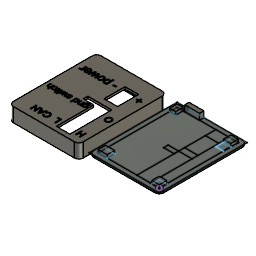
CANbuttonPresser (Autodesk Fusion 360 design; units mm, degrees)
Autodesk Fusion 360 part; units mm, degrees
sketch "Sketch1" plane through (0, 0, 0) normal (0, 0, 1) x (1, 0, 0)
  line L0 (0, 0) -> (-41, 0)
  line L1 (-41, 0) -> (-41, 53)
  line L2 (-41, 53) -> (0, 53)
  line L3 (0, 53) -> (0, 0)
  line L4 (-44, -3) -> (-44, 56)
  line L5 (-44, 56) -> (3, 56)
  line L6 (3, 56) -> (3, -3)
  line L7 (3, -3) -> (-44, -3)
  line L8 (-36, 53) -> (-26, 53)
  line L9 (-26, 53) -> (-26, 56)
  line L10 (-26, 56) -> (-36, 56)
  line L11 (-36, 56) -> (-36, 53)
  line L12 (-6, 53) -> (-6, 0)
  line L13 (-15, 53) -> (-15, 0)
  line L14 (-15, 28) -> (-22, 28)
  line L15 (-22, 28) -> (-22, 25)
  line L16 (-22, 25) -> (-15, 25)
  line L17 (-15, 25) -> (-15, 28) construction
  line L18 (-35, 0) -> (-41, 0)
  line L19 (-41, 0) -> (-41, 5)
  line L20 (-41, 5) -> (-35, 5)
  line L21 (-35, 5) -> (-35, 0)
  line L22 (-41, 53) -> (-37, 53)
  line L23 (-37, 53) -> (-37, 48)
  line L24 (-37, 48) -> (-41, 48)
  line L25 (-41, 48) -> (-41, 53)
  line L26 (0, 53) -> (-5, 53)
  line L27 (-5, 53) -> (-5, 48)
  line L28 (-5, 48) -> (0, 48)
  line L29 (0, 48) -> (0, 53)
  line L30 (0, 0) -> (-5, 0)
  line L31 (-5, 0) -> (-5, 5)
  line L32 (-5, 5) -> (0, 5)
  line L33 (0, 5) -> (0, 0)
  line L34 (-15, 46) -> (-6, 46)
  line L35 (-15, 28) -> (-6, 28)
  line L36 (-15, 32) -> (-6, 32)
  line L37 (-5, 48) -> (0, 48)
  line L38 (0, 48) -> (0, 43)
  line L39 (0, 43) -> (-5, 43)
  line L40 (-5, 43) -> (-5, 48)
  dimension "d1" = 53
  dimension "d2" = 41
  dimension "d3" = -3
  dimension "d4" = 10
  dimension "d5" = 5
  dimension "d6" = 6
  dimension "d7" = 9
  dimension "d8" = 25
  dimension "d9" = 7
  dimension "d10" = 3
  dimension "d21" = 7
  dimension "d32" = 4
  dimension "d41" = 4
  constraint horizontal L0
  constraint vertical L1
  constraint horizontal L2
  constraint vertical L3
  constraint coincident L0.start L3.end
  constraint horizontal L8
  constraint vertical L9
  constraint horizontal L10
  constraint vertical L11
  constraint coincident L2 L8.start
  constraint coincident L2 L12.start
  constraint coincident L0 L12.end
  constraint perpendicular L0 L12
  constraint coincident L2 L13.start
  constraint coincident L0 L13.end
  constraint perpendicular L0 L13
  constraint horizontal L14
  constraint vertical L15
  constraint horizontal L16
  constraint vertical L17
  constraint coincident L13 L14.start
  constraint horizontal L18
  constraint vertical L19
  constraint horizontal L20
  constraint vertical L21
  constraint coincident L1 L19.end
  constraint horizontal L22
  constraint vertical L23
  constraint horizontal L24
  constraint vertical L25
  constraint horizontal L26
  constraint vertical L27
  constraint horizontal L28
  constraint vertical L29
  constraint horizontal L30
  constraint vertical L31
  constraint horizontal L32
  constraint vertical L33
  constraint coincident L13 L34.start
  constraint coincident L12 L34.end
  constraint perpendicular L12 L34
  constraint coincident L12 L35.end
  constraint perpendicular L12 L35
  constraint coincident L13 L36.start
  constraint coincident L12 L36.end
  constraint perpendicular L12 L36
  constraint horizontal L37
  constraint vertical L38
  constraint horizontal L39
  constraint vertical L40
  constraint coincident L3 L38.end
  measures "d1" distance of L0.end L1.end
  measures "d2" distance of L0.start L0.end
  measures "d4" distance of L8.start L8.end
  measures "d5" distance of L1.end L11
  measures "d6" distance of L3 L12
  measures "d7" distance of L12 L13
  measures "d8" distance of L2 L14
  measures "d9" distance of L14.start L14.end
  measures "d10" distance of L14.end L15.end
  measures "d21" distance of L2 L34
  measures "d32" distance of L35 L36
  measures "d41" distance of L23.end L24.end
extrude "Extrude1" add sketch "Sketch1" along normal blind 1.5 contours L0 L1 L2 L3 L4 L5 L6 L7 L9 L11 L18 L19 L22 L25 L26 L29 L30 L33 L38 | L0 L3 L30 L31 L32 L33 | L0 L2 L3 L12 L27 L31 L32 L39 L40 | L3 L28 L37 L38 L39 L40 | L0 L1 L2 L8 L13 L14 L15 L16 L20 L21 L23 L24 | L12 L13 L35 L36 | L2 L3 L26 L27 L28 L29 L37 | L0 L1 L18 L19 L20 L21 | L2 L12 L13 L34 | L1 L2 L22 L23 L24 L25 | L2 L5 L8 L9 L10 L11 makes body 1
extrude "Extrude2" add sketch "Sketch1" against normal blind 8 contours L0 L1 L2 L3 L4 L5 L6 L7 L9 L11 L18 L19 L22 L25 L26 L29 L30 L33 L38 bodies 1
extrude "Extrude7" add sketch "Sketch1" against normal blind 3 contours L0 L3 L30 L31 L32 L33 | L3 L28 L37 L38 L39 L40 | L0 L1 L18 L19 L20 L21 bodies 1
move_body "Move1" bodies 1 to x (1, 0, 0) y (0, 1, 0) z (0, 0, 1) at (-54, 0, 0)
extrude "Extrude8" add sketch "Sketch1" against normal blind 1.2 separate body makes body 2
extrude "Extrude4" add sketch "Sketch1" along normal blind 2 and the other way blind 1 contours L0 L3 L30 L31 L32 L33 | L2 L3 L26 L27 L28 L29 L37 | L0 L1 L18 L19 L20 L21 | L1 L2 L22 L23 L24 L25 bodies 2
extrude "Extrude5" add sketch "Sketch1" along normal blind 4 contours L2 L5 L8 L9 L10 L11 bodies 2
fillet "Fillet1" radius 2 2 edges at (-80, 54.5, 0) (-90, 54.5, 0) on bodies 1
fillet "Fillet2" radius 3 8 edges at (-51, 56, -3.25) (-51, -3, -3.25) (-98, 56, -3.25) (-98, -3, -3.25) (3, -3, -0.6) (-44, -3, -0.6) (3, 56, -0.6) (-44, 56, -0.6) on bodies 1 2
sketch "Sketch2" plane through (0, 0, 1.5) normal (0, 0, 1) x (-1, 0, 0)
  arc A0 (98, 0) -> (95, 3) centre (95, 0) ccw
  line L0 (95, 3) -> (54, 3)
  arc A1 (54, 3) -> (51, 0) centre (54, 0) ccw
  line L1 (51, 0) -> (51, -53)
  arc A2 (51, -53) -> (54, -56) centre (54, -53) ccw
  line L2 (54, -56) -> (95, -56)
  arc A3 (95, -56) -> (98, -53) centre (95, -53) ccw
  line L3 (98, -53) -> (98, 0)
  line L4 (54.5628, -46.0404) -> (98.0169, -45.7556) construction
  line L5 (98.0169, -45.7556) -> (97.9831, -40.5942) construction
  line L6 (97.9831, -40.5942) -> (54.529, -40.8791) construction
  line L7 (54.529, -40.8791) -> (54.5628, -46.0404) construction
  line L8 (53.3651, -24.4416) -> (96.8192, -24.1567) construction
  line L9 (96.8192, -24.1567) -> (96.7854, -18.9954) construction
  line L10 (96.7854, -18.9954) -> (53.3313, -19.2803) construction
  line L11 (53.3313, -19.2803) -> (53.3651, -24.4416) construction
  line L12 (54.8378, -6.9343) -> (98.292, -6.6494) construction
  line L13 (98.292, -6.6494) -> (98.2581, -1.4881) construction
  line L14 (98.2581, -1.4881) -> (54.804, -1.773) construction
  line L15 (54.804, -1.773) -> (54.8378, -6.9343) construction
  line L16 (69, -32) -> (69, -46)
  line L17 (69, -46) -> (60, -46)
  line L18 (60, -46) -> (60, -32)
  line L19 (60, -32) -> (69, -32)
  line L20 (76, -25) -> (76, -28)
  line L21 (76, -28) -> (60, -28)
  line L22 (60, -28) -> (60, 0)
  line L23 (60, 0) -> (69, 0)
  line L24 (69, 0) -> (69, -25)
  line L25 (69, -25) -> (76, -25)
  dimension "d26" = 5
  dimension "d28" = 4
  dimension "d30" = 4
  text T0 "+       - power" font "Arial" height 5 align left top in box 43.4551 x 5.1614 at (54.5628, -46.0404) x (0.999979, 0.006555) y (-0.006555, 0.999979) spacing 1 kerned
  text T1 "O        gnd switch" font "Arial" height 4 align left top in box 43.4551 x 5.1614 at (53.3651, -24.4416) x (0.999979, 0.006555) y (-0.006555, 0.999979) spacing 1 kerned
  text T2 "H        L  CAN" font "Arial" height 4 align left top in box 43.4551 x 5.1614 at (54.8378, -6.9343) x (0.999979, 0.006555) y (-0.006555, 0.999979) spacing 1 kerned
  constraint coincident L3
extrude "Extrude6" cut sketch "Sketch2" against normal blind 0.4 text T2 T1 T0 bodies 1
equation "d27 = '+       - power'"
equation "d29 = 'O        gnd switch'"
equation "d31 = 'H        L  CAN'"
